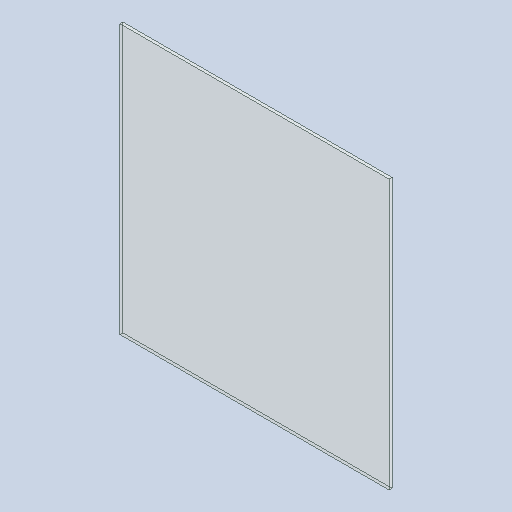
# Autodesk Inventor part: rectangle upper portion
Saved by Autodesk Inventor 2024 (Build 280153000, 153)
## iProperties
Created: 2023-06-03
Part Number: rectangle upper portion
Material: Glass
Document SubType Name: Modeling
Designer: Sahil Nadaf
Density: 2.18 g/cm^3
Appearance: Clear
Author: Sahil Nadaf
Autodesk Inventor part; units mm, degrees
ref_plane "YZ Plane" through (0, 0, 0) normal (1, 0, 0) x (0, 1, 0)
ref_plane "XZ Plane" through (0, 0, 0) normal (0, 1, 0) x (-1, 0, 0)
ref_plane "XY Plane" through (0, 0, 0) normal (0, 0, 1) x (1, 0, 0)
sketch "Sketch1" plane through (0, 0, 0) normal (0, 0, 1) x (1, 0, 0)
  line L0 (-27.5149, 11.9796) -> (429.4851, 11.9796)
  line L1 (429.4851, 11.9796) -> (429.4851, -445.0204)
  line L2 (429.4851, -445.0204) -> (-27.5149, -445.0204)
  line L3 (-27.5149, -445.0204) -> (-27.5149, 11.9796)
  point P0 (0, 0)
  dimension "d0" = 457
  dimension "d1" = 457
  constraints: 8 end point, 2 parallel, 1 horizontal, 1 perpendicular
  measures "d0" distance of L1.end L2.end
  measures "d1" distance of L0.end L1.end
extrude "Extrusion1" add sketch "Sketch1" along normal blind 5
body "Solid1"
